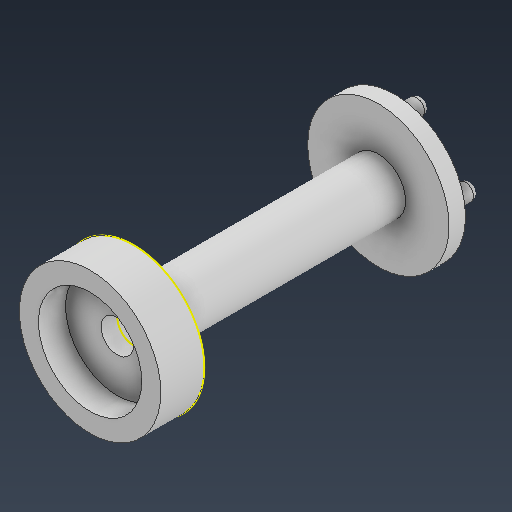
# Autodesk Inventor part: вт1
Saved by Autodesk Inventor 2025 (Build 290162000, 162)
## iProperties
Created: 2025-03-14
Part Number: вт1
Material: Типовые
Document SubType Name: Modeling
Designer: GameHD
Density: 1 g/cm^3
Appearance: По умолчанию
Author: GameHD
Autodesk Inventor part; units mm, degrees
ref_plane "YZ Plane" through (0, 0, 0) normal (1, 0, 0) x (0, 1, 0)
ref_plane "XZ Plane" through (0, 0, 0) normal (0, 1, 0) x (-1, 0, 0)
ref_plane "XY Plane" through (0, 0, 0) normal (0, 0, 1) x (1, 0, 0)
sketch "Эскиз1" plane through (0, 0, 0) normal (0, 0, 1) x (1, 0, 0)
  circle A0 centre (0, 0) radius 3
  circle A1 centre (0, 0) radius 5
  dimension "d0" = 6
  dimension "d1" = 10
  constraints: 2 centre point, 2 coincident
  measures "d0" diameter of A0
  measures "d1" diameter of A1
extrude "Выдавливание1" add sketch "Эскиз1" along normal blind 45
sketch "Эскиз2" plane through (0, 0, 0) normal (0, 0, -1) x (-1, 0, 0)
  circle A0 centre (0, 0) radius 13
  circle A1 centre (0, 0) radius 5 projected
  circle A2 centre (0, 0) radius 3 projected
  dimension "d4" = 26
  constraints: 1 centre point, 1 coincident
  measures "d4" diameter of A0
extrude "Выдавливание2" add sketch "Эскиз2" along normal blind 3 contours A0 | A1
sketch "Эскиз3" plane through (0, 0, -3) normal (0, 0, -1) x (-1, 0, 0)
  circle A0 centre (0, 9) radius 1.5
  circle A1 centre (-9, 0) radius 1.5
  circle A2 centre (0, -9) radius 1.5
  circle A3 centre (9, 0) radius 1.5
  circle A4 centre (0, 0) radius 5 projected
  dimension "d7" = 3
  dimension "d8" = 3
  dimension "d10" = 3
  dimension "d23" = 3
  dimension "d24" = 9
  dimension "d25" = 9
  dimension "d26" = 9
  dimension "d27" = 9
  constraints: 4 centre point
  measures "d7" diameter of A0
  measures "d8" diameter of A1
  measures "d10" diameter of A2
  measures "d23" diameter of A3
  measures "d24" distance of A3.centre point (0, 0)
  measures "d25" distance of A0.centre point (0, 0)
  measures "d26" distance of A4.centre A2.centre
  measures "d27" distance of A1.centre point (0, 0)
extrude "Выдавливание3" add sketch "Эскиз3" along normal blind 5 contours A0 | A1 | A2 | A3
fillet "Сопряжение1" radius 1 4 edges at (1.5, 9, -8) (10.5, 0, -8) (1.5, -9, -8) (-7.5, 0, -8)
sketch "Эскиз4" plane through (0, 0, 45) normal (0, 0, 1) x (1, 0, 0)
  circle A0 centre (0, 9) radius 1.5 projected
  circle A1 centre (0, 0) radius 13 projected
  circle A2 centre (0, 0) radius 5 projected
  circle A3 centre (0, 0) radius 3 projected
  point P0 (-0.5792, 4.9663)
  point P1 (0.5792, 4.9663)
extrude "Выдавливание4" add sketch "Эскиз4" along normal blind 3 contours A0 | A1 | A2
sketch "Эскиз6" plane through (0, 0, 48) normal (0, 0, 1) x (1, 0, 0)
  circle A0 centre (0, 0) radius 9.5
  circle A1 centre (0, 0) radius 13 projected
  dimension "d19" = 19
  constraints: 1 centre point
  measures "d19" diameter of A0
extrude "Выдавливание6" add sketch "Эскиз6" along normal blind 5
